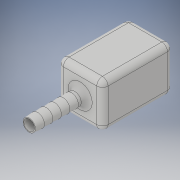
# Autodesk Inventor part: Square-Circle-Adapter V1D1-OUT
Saved by Autodesk Inventor 2017 (Build 210142000, 142)
## iProperties
Created: 2017-12-22
Part Number: Square-Circle-Adapter V1D1-OUT
Material: Generic
Document SubType Name: Modeling
Designer: Tripl_000
Density: 1 g/cm^3
Appearance: Default
Author: Tripl_000
Autodesk Inventor part; units mm, degrees
ref_plane "YZ Plane" through (0, 0, 0) normal (1, 0, 0) x (0, 1, 0)
ref_plane "XZ Plane" through (0, 0, 0) normal (0, 1, 0) x (-1, 0, 0)
ref_plane "XY Plane" through (0, 0, 0) normal (0, 0, 1) x (1, 0, 0)
sketch "Sketch1" plane through (0, 0, 0) normal (0, 0, 1) x (1, 0, 0)
  line L0 (-7.9, 7.9) -> (7.9, 7.9)
  line L1 (7.9, 7.9) -> (7.9, -7.9)
  line L2 (7.9, -7.9) -> (-7.9, -7.9)
  line L3 (-7.9, -7.9) -> (-7.9, 7.9)
  line L4 (-7.9, 7.9) -> (7.9, -7.9) construction
  line L5 (7.9, 7.9) -> (-7.9, -7.9) construction
  point P0 (0, 0)
  dimension "d0" = 15.8
  dimension "d1" = 15.8
  constraints: 12 end point, 2 midpoint, 2 parallel, 1 horizontal, 1 perpendicular
  measures "d0" distance of L2.end L0.start
  measures "d1" distance of L0.start L0.end
extrude "Extrusion1" add sketch "Sketch1" along normal blind 15
sketch "Sketch2" plane through (0, 0, 15) normal (0, 0, 1) x (1, 0, 0)
  line L0 (-6.4, 6.4) -> (6.4, 6.4)
  line L1 (6.4, 6.4) -> (6.4, -6.4)
  line L2 (6.4, -6.4) -> (-6.4, -6.4)
  line L3 (-6.4, -6.4) -> (-6.4, 6.4)
  line L4 (-6.4, 6.4) -> (6.4, -6.4) construction
  line L5 (6.4, 6.4) -> (-6.4, -6.4) construction
  point P0 (0, 0)
  dimension "d4" = 12.8
  dimension "d5" = 12.8
  constraints: 12 end point, 2 midpoint, 2 parallel, 1 horizontal, 1 perpendicular
  measures "d4" distance of L0.end L1.end
  measures "d5" distance of L0.start L0.end
extrude "Extrusion2" cut sketch "Sketch2" against normal through all
sketch "Sketch5" plane through (0, 0, 15) normal (0, 0, 1) x (1, 0, 0)
  line L0 (7.9, 7.9) -> (-7.9, 7.9) projected
  line L1 (7.9, 7.9) -> (7.9, -7.9) projected
  line L2 (-7.9, 7.9) -> (7.9, 7.9)
  line L3 (7.9, 7.9) -> (7.9, -7.9)
  line L4 (7.9, -7.9) -> (-7.9, -7.9)
  line L5 (-7.9, -7.9) -> (-7.9, 7.9)
  point P0 (0, 0)
  constraints: 8 end point, 2 parallel, 1 horizontal, 1 perpendicular
extrude "Extrusion5" add sketch "Sketch5" along normal blind 10
ref_plane "Work Plane2" through (0, -7.9, 0) normal (1, 0, 0) x (0, 0, -1)
sketch "Sketch6" plane through (0, -7.9, 0) normal (1, 0, 0) x (0, 0, -1)
  line L0 (-7.1534, 7.9) -> (-46.3689, 7.9)
  line L1 (-25, 15.8) -> (-25, 0) projected
  line L2 (-25, 7.9) -> (-25, 10.3)
  line L3 (-25, 10.3) -> (-28, 10.1)
  line L4 (-28, 10.1) -> (-28, 7.9)
  line L5 (-28, 10.1) -> (-28, 10.3)
  line L6 (-28, 10.3) -> (-31, 10.1)
  line L7 (-31, 10.1) -> (-31, 7.9)
  line L8 (-31, 10.1) -> (-31, 10.3)
  line L9 (-31, 10.3) -> (-34, 10.1)
  line L10 (-34, 10.1) -> (-34, 7.9)
  line L11 (-34, 10.1) -> (-34, 10.3)
  line L12 (-34, 10.3) -> (-37, 10.1)
  line L13 (-37, 10.1) -> (-37, 7.9)
  line L14 (-37, 10.1) -> (-37, 10.3)
  line L15 (-37, 10.3) -> (-40, 10.1)
  line L16 (-40, 10.1) -> (-40, 7.9)
  line L17 (-40, 10.1) -> (-40, 10.3)
  line L18 (-40, 10.3) -> (-42.9988, 10.1)
  line L19 (-42.9988, 10.1) -> (-42.9988, 7.9)
  line L20 (-28, 7.9) -> (-25, 7.9)
  line L21 (-25, 10.3) -> (-25, 7.9)
  line L22 (-25, 10.3) -> (-28, 10.1)
  line L23 (-28, 10.1) -> (-28, 7.9)
  point P0 (0, 7.9)
  dimension "d23" = 2.4
  dimension "d24" = 0.2
  dimension "d25" = 0
  dimension "d26" = 3
  dimension "d27" = 3
  dimension "d28" = 3
  dimension "d29" = 3
  dimension "d30" = 3
  dimension "d31" = 2.4
  dimension "d32" = 2.4
  dimension "d33" = 2.4
  dimension "d34" = 2.2
  dimension "d35" = 2.2
  constraints: 46 end point, 7 point on line, 6 perpendicular, 5 vertical, 3 parallel, 1 collinear, 1 horizontal, 1 midpoint
  measures "d23" distance of L2.end L2.start
  measures "d24" vertical distance of L2.end L3.end
  measures "d25" distance from line of L2.start L0
  measures "d26" distance between parallel lines of L1 L4
  measures "d27" distance from line of L4 L6.end
  measures "d28" distance between parallel lines of L17 L14
  measures "d29" distance between parallel lines of L11 L14
  measures "d30" distance between parallel lines of L8 L11
  measures "d31" distance of L5.end L4.end
  measures "d32" distance of L13.end L14.end
  measures "d33" distance of L16.end L17.end
  measures "d34" distance from line of L0 L6.end
  measures "d35" distance of L18.end L19.end
revolve "Revolution1" add sketch "Sketch6" angle 360 about axis through (0, 0, 7.1534) along (0, 0, 1)
sketch "Sketch7" plane through (0, 0, 42.9988) normal (0, 0, 1) x (1, 0, 0)
  circle A0 centre (0, 0) radius 1.9
  dimension "d37" = 3.8
  constraints: 1 centre point, 1 coincident
  measures "d37" diameter of A0
extrude "Extrusion6" cut sketch "Sketch7" against normal through all
fillet "Fillet4" radius 2 8 edges at (6.4, -6.4, 7.5) (-6.4, -6.4, 7.5) (-6.4, 6.4, 7.5) (6.4, 6.4, 7.5) (-7.9, 7.9, 12.5) (7.9, 7.9, 12.5) (7.9, -7.9, 12.5) (-7.9, -7.9, 12.5)
fillet "Fillet5" radius 2 9 edges at (-1.9, 0, 15) (-5.8142, -5.8142, 15) (-6.4, 0, 15) (-5.8142, 5.8142, 15) (0, 6.4, 15) (5.8142, 5.8142, 15) (6.4, 0, 15) (5.8142, -5.8142, 15) (0, -6.4, 15)
fillet "Fillet6" radius 2 16 edges at (7.3142, 7.3142, 25) (0, 7.9, 25) (-7.3142, 7.3142, 25) (-7.9, 0, 25) (-7.3142, -7.3142, 25) (0, -7.9, 25) (7.3142, -7.3142, 25) (7.9, 0, 25) (7.3142, -7.3142, 0) (0, -7.9, 0) (-7.3142, -7.3142, 0) (-7.9, 0, 0) (-7.3142, 7.3142, 0) (0, 7.9, 0) (7.3142, 7.3142, 0) (7.9, 0, 0)
fillet "Fillet7" radius 2 1 edges at (0, -2.4, 25)
body "Solid1"
